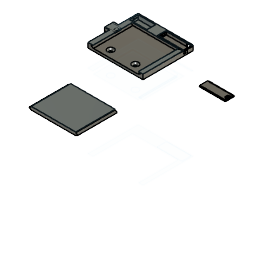
3d molde Home assistnt tablat (Autodesk Fusion 360 design; units mm, degrees)
part number: 2026-03-25-17-44-52-622
Autodesk Fusion 360 part; units mm, degrees
note: some values were not read from the file. Chosen so that the rebuilt part matches the saved one: which bodies a step acts on; which face or edge a step refers to.
(part 1 of 2)
sketch "Skizze1" plane through (0, 0, 0) normal (0, 0, 1) x (1, 0, 0)
  line L0 (0, 0) -> (242, 0)
  line L1 (242, 0) -> (242, 166)
  line L2 (242, 166) -> (0, 166)
  line L3 (0, 166) -> (0, 0)
  dimension "d1" = 242
  dimension "d2" = 166
  constraint horizontal L0
  constraint vertical L1
  constraint horizontal L2
  constraint vertical L3
  constraint coincident L0.start L3.end
  measures "d1" distance of L0.start L0.end
  measures "d2" distance of L0.start L2.end
extrude "Extrusion1" add sketch "Skizze1" along normal blind 7.5 makes body 1
fillet "Abrundung1" radius 7.5 4 edges at (0, 0, 3.75) (242, 0, 3.75) (242, 166, 3.75) (0, 166, 3.75) on bodies 1
sketch "Skizze2" plane through (0, 0, 7.5) normal (0, 0, 1) x (-1, 0, 0)
  arc A0 (-7.5, -166) -> (0, -158.5) centre (-7.5, -158.5) ccw
  line L0 (0, -158.5) -> (0, -7.5)
  arc A1 (0, -7.5) -> (-7.5, 0) centre (-7.5, -7.5) ccw
  line L1 (-7.5, 0) -> (-234.5, 0)
  arc A2 (-234.5, 0) -> (-242, -7.5) centre (-234.5, -7.5) ccw
  line L2 (-242, -7.5) -> (-242, -158.5)
  arc A3 (-242, -158.5) -> (-234.5, -166) centre (-234.5, -158.5) ccw
  line L3 (-234.5, -166) -> (-7.5, -166)
  line L4 (-199.0459, -30) -> (-43.7756, -30)
  line L5 (-43.7756, -30) -> (-43.7756, -136.2508)
  line L6 (-43.7756, -136.2508) -> (-199.0459, -136.2508)
  line L7 (-199.0459, -136.2508) -> (-199.0459, -30)
  constraint horizontal L4
  constraint vertical L5
  constraint horizontal L6
  constraint vertical L7
extrude "Extrusion2" add sketch "Skizze2" along normal blind 10 contours L4 L5 L6 L7 bodies 1
sketch "Skizze3" plane through (0, 166, 0) normal (0, 1, 0) x (-1, 0, 0)
  line L0 (-7.5, 0) -> (-7.5, 7.5)
  line L1 (-7.5, 7.5) -> (-234.5, 7.5)
  line L2 (-234.5, 7.5) -> (-234.5, 0)
  line L3 (-234.5, 0) -> (-7.5, 0)
  line L4 (-259.0579, 7.5) -> (20, 7.5)
  line L5 (20, 7.5) -> (20, -40)
  line L6 (20, -40) -> (-259.0579, -40)
  line L7 (-259.0579, -40) -> (-259.0579, 7.5)
  constraint horizontal L4
  constraint vertical L5
  constraint horizontal L6
  constraint vertical L7
extrude "Extrusion3" cut sketch "Skizze3" against normal blind 170 bodies 1
sketch "Skizze4" plane through (0, 0, 17.5) normal (0, 0, 1) x (-1, 0, 0)
  line L0 (-199.0459, -136.2508) -> (-43.7756, -136.2508)
  line L1 (-43.7756, -136.2508) -> (-43.7756, -30)
  line L2 (-43.7756, -30) -> (-199.0459, -30)
  line L3 (-199.0459, -30) -> (-199.0459, -136.2508)
  line L4 (40, -30) -> (140, -30)
  line L5 (140, -30) -> (140, -110)
  line L6 (140, -110) -> (40, -110)
  line L7 (40, -110) -> (40, -30)
  dimension "d15" = 100
  dimension "d16" = 80
  constraint horizontal L4
  constraint vertical L5
  constraint horizontal L6
  constraint vertical L7
  measures "d15" distance of L4.start L4.end
  measures "d16" distance of L4.start L6.end
extrude "Extrusion4" add sketch "Skizze4" against normal blind 5 separate body contours L4 L5 L6 L7 makes body 2
extrude "Extrusion5" add 1 faces at (-73.3333, 56.6667, 17.5) along direction (0, 0, 1) blind 10 on bodies 2 bodies 2
sketch "Skizze5" plane through (0, 0, 27.5) normal (0, 0, 1) x (-1, 0, 0)
  line L0 (40, -110) -> (140, -110)
  line L1 (140, -110) -> (140, -30)
  line L2 (140, -30) -> (40, -30)
  line L3 (40, -30) -> (40, -110)
extrude "Extrusion6" cut sketch "Skizze5" against normal blind 10 bodies 2
extrude "Extrusion7" add 1 faces at (-73.3333, 56.6667, 17.5) along direction (0, 0, 1) blind 0.5 on bodies 2 bodies 2
sketch "Skizze6" plane through (0, 30, 0) normal (0, -1, 0) x (1, 0, 0)
  line L0 (-140, 18) -> (-140, 12.5)
  line L1 (-140, 12.5) -> (-40, 12.5)
  line L2 (-40, 12.5) -> (-40, 18)
  line L3 (-40, 18) -> (-140, 18)
  line L4 (-140, 15.25) -> (-134.9888, 18)
  line L5 (-140, 18) -> (-140, 12.5)
  line L6 (-135.0937, 12.5) -> (-140, 15.25)
  line L7 (-140, 12.5) -> (-135.0937, 12.5)
  line L8 (-140, 18) -> (-134.9888, 18)
  line L9 (-44.7811, 18) -> (-40, 15.25)
  line L10 (-44.886, 12.5) -> (-40, 15.25)
  line L11 (-44.886, 12.5) -> (-40, 12.5)
  line L12 (-40, 12.5) -> (-40, 18)
  line L13 (-40, 18) -> (-44.7811, 18)
  constraint midpoint L0 L4.start
  constraint coincident L3 L4.end
  constraint coincident L0.start L3.end
  constraint coincident L0.end L1.start
  constraint coincident L1 L6.start
  constraint coincident L3 L9.start
  constraint midpoint L2 L9.end
  constraint coincident L1 L10.start
  constraint coincident L1.end L2.start
  constraint coincident L2.end L3.start
extrude "Extrusion8" cut sketch "Skizze6" against normal blind 90 contours L0 L3 L4 L5 L8 | L0 L1 L5 L6 L7 | L2 L3 L9 L12 L13 | L1 L2 L10 L11 L12 bodies 2
move_body "Verschieben1" bodies 2 to x (1, 0, 0) y (0, 1, 0) z (0, 0, 1) at (210, -110, 0)
move_body "Verschieben2" bodies 2 to x (1, 0, 0) y (0, 1, 0) z (0, 0, 1) at (-10, 0, 0)
sketch "Skizze7" plane through (0, 0, 17.5) normal (0, 0, 1) x (-1, 0, 0)
  line L0 (-199.0459, -136.2508) -> (-43.7756, -136.2508)
  line L1 (-43.7756, -136.2508) -> (-43.7756, -30)
  line L2 (-43.7756, -30) -> (-199.0459, -30)
  line L3 (-199.0459, -30) -> (-199.0459, -136.2508)
  line L4 (-175.238, -30) -> (-199.0459, -30)
  line L5 (-199.0459, -136.2508) -> (-175, -136.2508)
  line L6 (-175.238, -30) -> (-175, -136.2508)
  line L7 (-199.0459, -30) -> (-199.0459, -136.2508)
  constraint coincident L2 L4.start
  constraint coincident L2.end L3.start
  constraint coincident L0.start L3.end
  constraint coincident L0 L5.end
extrude "Extrusion9" cut sketch "Skizze7" against normal blind 150 contours L0 L2 L3 L4 L5 L6 L7 bodies 1
sketch "Skizze8" plane through (0, 0, 17.5) normal (0, 0, 1) x (-1, 0, 0)
  line L0 (-175.238, -30) -> (-175, -136.2508)
  line L1 (-175, -136.2508) -> (-43.7756, -136.2508)
  line L2 (-43.7756, -136.2508) -> (-43.7756, -30)
  line L3 (-43.7756, -30) -> (-175.238, -30)
  line L4 (-180, -130) -> (-40, -130)
  line L5 (-40, -130) -> (-40, -140)
  line L6 (-40, -140) -> (-180, -140)
  line L7 (-180, -140) -> (-180, -130)
  constraint horizontal L4
  constraint vertical L5
  constraint horizontal L6
  constraint vertical L7
extrude "Extrusion10" cut sketch "Skizze8" against normal blind 20 contours L0 L1 L2 L4 | L0 L1 L2 L4 L5 L6 L7 bodies 1
extrude "Extrusion11" cut 1 faces at (95.0105, 0, 14.3333) along direction (0, 1, 0) blind 120 on bodies 2 bodies 1
move_body "Verschieben3" bodies 2 to x (1, 0, 0) y (0, 1, 0) z (0, 0, 1) at (0, 25, 0)
sketch "Skizze9" plane through (0, 0, 12.5) normal (0, 0, 1) x (-1, 0, 0)
  line L0 (-64.9063, -30) -> (-155.114, -30)
  line L1 (-155.114, -30) -> (-155.114, -120)
  line L2 (-155.114, -120) -> (-64.9063, -120)
  line L3 (-64.9063, -120) -> (-64.9063, -30)
  line L4 (-135, -45) -> (-175, -45)
  line L5 (-45, -45) -> (-85, -45)
  dimension "d33" = 40
  constraint perpendicular L3 L5
  constraint horizontal L4
  measures "d33" distance of L5.start L5.end
hole "Bohrung1" at (85, 45, 12.5) at (135, 45, 12.5) direction (0, 0, -1) diameter 6 depth 55 tip angle 118 countersink diameter 13 countersink angle 90 bodies 1
extrude "Extrusion12" add 1 faces at (125.1008, 120, 15.8333) along direction (0, -1, 0) blind 10 on bodies 1 bodies 1
move_body "Verschieben4" bodies 2 to x (1, 0, 0) y (0, 1, 0) z (0, 0, 1) at (0, 0, -50)
extrude "Extrusion13" cut 1 faces at (87.5217, 130, 10.8333) along direction (0, -1, 0) blind 10 on bodies 1 bodies 1
extrude "Extrusion14" cut 1 faces at (175.1633, 63.3333, 14.1667) along direction (-0.999997, -0.00224, 0) blind 10 on bodies 1 bodies 1
extrude "Extrusion15" cut 1 faces at (43.7756, 60, 10.8333) along direction (1, 0, 0) blind 10 on bodies 1 bodies 1
move_body "Verschieben5" bodies 2 to x (1, 0, 0) y (0, 1, 0) z (0, 0, 1) at (0, -20, 50)
extrude "Extrusion16" add 1 faces at (127.9494, 120, 10.8333) along direction (0, 1, 0) blind 10 on bodies 1 bodies 1
sketch "Skizze10" plane through (0, 0, 17.5) normal (0, 0, 1) x (-1, 0, 0)
extrude "Extrusion17" add 1 faces at (127.9494, 130, 10.8333) along direction (0, 1, 0) blind 2 on bodies 1 bodies 1
sketch "Skizze11" plane through (0, 0, 17.5) normal (0, 0, 1) x (-1, 0, 0)
  line L0 (-162.2484, -111.5795) -> (-132.2484, -111.5795)
  line L1 (-132.2484, -111.5795) -> (-132.2484, -130.0795)
  line L2 (-132.2484, -130.0795) -> (-162.2484, -130.0795)
  line L3 (-162.2484, -130.0795) -> (-162.2484, -111.5795)
  dimension "d51" = 30
  dimension "d52" = 18.5
  constraint horizontal L0
  constraint vertical L1
  constraint horizontal L2
  constraint vertical L3
  measures "d51" distance of L0.start L0.end
  measures "d52" distance of L0.start L2.end
sketch "Skizze12" plane through (0, 0, 17.5) normal (0, 0, 1) x (-1, 0, 0)
extrude "Extrusion18" cut sketch "Skizze11" against normal blind 8 bodies 1
sketch "Skizze13" plane through (0, 132, 0) normal (0, 1, 0) x (-1, 0, 0)
  line L0 (-53.7756, 7.5) -> (-53.7756, 17.5)
  line L1 (-53.7756, 17.5) -> (-165.0364, 17.5)
  line L2 (-165.0364, 17.5) -> (-165.0364, 7.5)
  line L3 (-165.0364, 7.5) -> (-53.7756, 7.5)
  line L4 (-162, 15) -> (-153, 15)
  line L5 (-153, 15) -> (-153, 12)
  line L6 (-153, 12) -> (-162, 12)
  line L7 (-162, 12) -> (-162, 15)
  dimension "d55" = 9
  dimension "d56" = 3
  constraint horizontal L4
  constraint vertical L5
  constraint horizontal L6
  constraint vertical L7
  measures "d55" distance of L4.start L4.end
  measures "d56" distance of L4.start L6.end
extrude "Extrusion19" cut sketch "Skizze13" against normal blind 5 contours L4 L5 L6 L7 bodies 1
extrude "Extrusion20" cut 1 faces at (156, 131.3598, 12) along direction (0, 0, -1) blind 3 on bodies 1 bodies 1
extrude "Extrusion21" add 1 faces at (125.1497, -48.3333, 18) along direction (0, 0, 1) blind 1 on bodies 2 bodies 2
extrude "Extrusion22" cut 1 faces at (156.8126, -48.3333, 17.0833) along direction (-0.498592, 0, -0.866837) blind 0.2 on bodies 2 bodies 2
extrude "Extrusion23" cut 1 faces at (156.6751, -21.6667, 13.3786) along direction (-0.490484, 0, 0.87145) blind 0.2 on bodies 2 bodies 2
extrude "Extrusion24" cut 1 faces at (63.2709, -48.3333, 13.4167) along direction (0.488937, 0, 0.872319) blind 0.2 on bodies 2 bodies 2
extrude "Extrusion25" cut 1 faces at (63.4097, -21.6667, 17.1211) along direction (0.481091, 0, -0.876671) blind 0.2 on bodies 2 bodies 2
sketch "Skizze14" plane through (0, 0, 19) normal (0, 0, 1) x (-1, 0, 0)
  line L0 (-155.2189, 75) -> (-155.2189, -5)
  line L1 (-155.2189, -5) -> (-65.0112, -5)
  line L2 (-65.0112, -5) -> (-65.0112, 75)
  line L3 (-65.0112, 75) -> (-155.2189, 75)
  line L4 (-4.4649, 104.0889) -> (237.5351, 104.0889)
  line L5 (237.5351, 104.0889) -> (237.5351, -61.9111)
  line L6 (237.5351, -61.9111) -> (-4.4649, -61.9111)
  line L7 (-4.4649, -61.9111) -> (-4.4649, 104.0889)
  dimension "d71" = 242
  dimension "d72" = 166
  constraint horizontal L4
  constraint vertical L5
  constraint horizontal L6
  constraint vertical L7
  measures "d71" distance of L4.start L4.end
  measures "d72" distance of L4.start L6.end
sketch "Skizze15" plane through (0, 0, 26.7) normal (0, 0, 1) x (-1, 0, 0)
  arc A0 (3.0351, 104.0889) -> (-4.4649, 96.5889) centre (3.0351, 96.5889) ccw
  line L0 (-4.4649, 96.5889) -> (-4.4649, -54.4111)
  arc A1 (-4.4649, -54.4111) -> (3.0351, -61.9111) centre (3.0351, -54.4111) ccw
  line L1 (3.0351, -61.9111) -> (230.0351, -61.9111)
  arc A2 (230.0351, -61.9111) -> (237.5351, -54.4111) centre (230.0351, -54.4111) ccw
  line L2 (237.5351, -54.4111) -> (237.5351, 96.5889)
  arc A3 (237.5351, 96.5889) -> (230.0351, 104.0889) centre (230.0351, 96.5889) ccw
  line L3 (230.0351, 104.0889) -> (3.0351, 104.0889)
  line L4 (9.6749, 27.3289) -> (3.4349, 27.3289)
  line L5 (3.4349, 27.3289) -> (3.4351, 21.0889)
  line L6 (9.6749, 27.3289) -> (15.9149, 27.3289)
  line L7 (15.9149, 27.3289) -> (15.9149, 14.8489)
  line L8 (15.9149, 14.8489) -> (3.4349, 14.8485)
  line L9 (3.4349, 14.8485) -> (3.4349, 27.3289)
  dimension "d80" = 6.24
  dimension "d81" = 6.24
  dimension "d82" = 12.48
  constraint perpendicular L4 L7
  constraint perpendicular L5 L8
  constraint perpendicular L4 L9
  measures "d80" distance of L4.start L4.end
  measures "d81" distance of L4.start L6.end
  measures "d82" distance of L6.end L7.end
sketch "Skizze16" plane through (0, 0, 27.2) normal (0, 0, 1) x (-1, 0, 0)
  line L0 (15.4149, 15.3489) -> (15.4149, 26.8289)
  line L1 (15.4149, 26.8289) -> (3.9349, 26.8289)
  line L2 (3.9349, 26.8289) -> (3.9349, 15.3485)
  line L3 (3.9349, 15.3485) -> (15.4149, 15.3489)
  circle A0 centre (9.6749, 21.0887) radius 1.75
  dimension "d87" = 3.5
  measures "d87" diameter of A0
sketch "Skizze17" plane through (-237.5351, 0, 0) normal (-1, 0, 0) x (0, -1, 0)
  line L0 (96.5889, 19) -> (96.5889, 26.7)
  line L1 (96.5889, 26.7) -> (-54.4111, 26.7)
  line L2 (-54.4111, 26.7) -> (-54.4111, 19)
  line L3 (-54.4111, 19) -> (96.5889, 19)
  line L4 (18.0776, 22.85) -> (18.0776, 21.5)
  line L5 (23.9968, 22.85) -> (24, 21.5)
  line L6 (23.9968, 22.85) -> (23.7, 23.2)
  line L7 (18.0776, 22.85) -> (18.4903, 23.2)
  line L8 (21.0889, 23.2) -> (23.7, 23.2)
  line L9 (18.4903, 23.2) -> (21.0889, 23.2)
  line L10 (18.0776, 21.5) -> (24, 21.5)
  constraint perpendicular L6 L7
sketch "Skizze18" plane through (-232.5351, 0, 0) normal (-1, 0, 0) x (0, -1, 0)
  line L0 (18.0776, 22.85) -> (18.0776, 21.5)
  line L1 (18.0776, 21.5) -> (24, 21.5)
  line L2 (24, 21.5) -> (23.9968, 22.85)
  line L3 (23.9968, 22.85) -> (23.7, 23.2)
  line L4 (23.7, 23.2) -> (21.0889, 23.2)
  line L5 (21.0889, 23.2) -> (18.4903, 23.2)
  line L6 (18.4903, 23.2) -> (18.0776, 22.85)
  line L7 (19, 22.5) -> (23, 22.5)
  line L8 (23, 22.5) -> (23, 22)
  line L9 (23, 22) -> (19, 22)
  line L10 (19, 22) -> (19, 22.5)
  constraint horizontal L7
  constraint vertical L8
  constraint horizontal L9
  constraint vertical L10
move_body "Verschieben6" bodies 2 to x (1, 0, 0) y (0, 1, 0) z (0, 0, 1) at (-225, 10, 25)
move_body "Verschieben7" bodies 2 to x (1, 0, 0) y (0, 1, 0) z (0, 0, 1) at (0, 5, 0)
sketch "Skizze19" plane through (0, 0, 44) normal (0, 0, 1) x (-1, 0, 0)
move_body "Verschieben8" [no effect]
move_body "Verschieben9" bodies 1 to x (1, 0, 0) y (0, 1, 0) z (0, 0, 1) at (-75, 0, 0)
move_body "Verschieben10" bodies 1 to x (1, 0, 0) y (0, 1, 0) z (0, 0, 1) at (-140, 0, 50)
move_body "Verschieben11" bodies 1 to x (1, 0, 0) y (0, 1, 0) z (0, 0, 1) at (120, 0, -70)
move_body "Verschieben12" bodies 2 to x (1, 0, 0) y (0, 1, 0) z (0, 0, 1) at (135, 14, -50)
move_body "Verschieben13" bodies 2 to x (1, 0, 0) y (0, 1, 0) z (0, 0, 1) at (-5, 0, 5)
extrude "Extrusion31" cut 1 faces at (37.2484, 117.7462, -5.1667) along direction (-1, 0, 0) blind 20 on bodies 1 bodies 1
extrude "Extrusion32" cut 1 faces at (30.8322, 130.0795, -6) along direction (0, 1, 0) blind 0.5 on bodies 1 bodies 1
move_body "Verschieben14" bodies 2 to x (1, 0, 0) y (0, 1, 0) z (0, 0, 1) at (0, -50, 0)
sketch "Skizze20" plane through (17.2484, 0, 0) normal (1, 0, 0) x (0, 1, 0)
  line L0 (130.5795, -2.5) -> (111.5795, -2.5)
  line L1 (111.5795, -2.5) -> (111.5795, -10.5)
  line L2 (111.5795, -10.5) -> (130.5795, -10.5)
  line L3 (130.5795, -10.5) -> (130.5795, -2.5)
  circle A0 centre (121.0795, -6.5) radius 1.5
  dimension "d106" = 3
  measures "d106" diameter of A0
sketch "Skizze21" plane through (0, 0, -2.5) normal (0, 0, 1) x (-1, 0, 0)
  line L0 (41.2244, -132) -> (41.2244, -30)
  line L1 (41.2244, -30) -> (30.8999, -30)
  line L2 (30.8999, -30) -> (30.8999, -110)
  line L3 (30.8999, -110) -> (-61.0882, -110)
  line L4 (-61.0882, -110) -> (-61.0882, -30)
  line L5 (-61.0882, -30) -> (-70.2379, -30)
  line L6 (-70.2379, -30) -> (-70.0364, -120)
  line L7 (-70.0364, -120) -> (-70.0364, -132)
  line L8 (-70.0364, -132) -> (41.2244, -132)
  line L9 (-17.2484, -111.5795) -> (-17.2484, -130.5795)
  line L10 (-17.2484, -130.5795) -> (-67.2484, -130.5795)
  line L11 (-67.2484, -130.5795) -> (-67.2484, -111.5795)
  line L12 (-67.2484, -111.5795) -> (-17.2484, -111.5795)
sketch "Skizze22" plane through (0, 30, 0) normal (0, -1, 0) x (1, 0, 0)
  line L0 (-41.2244, -2.5) -> (-41.2244, -12.5)
  line L1 (-41.2244, -12.5) -> (70.2379, -12.5)
  line L2 (70.2379, -12.5) -> (70.2379, -2.5)
  line L3 (70.2379, -2.5) -> (61.0882, -2.5)
  line L4 (61.0882, -2.5) -> (65, -4.75)
  line L5 (65, -4.75) -> (60.114, -7.5)
  line L6 (60.114, -7.5) -> (-30.0937, -7.5)
  line L7 (-30.0937, -7.5) -> (-35, -4.75)
  line L8 (-35, -4.75) -> (-30.8999, -2.5)
  line L9 (-30.8999, -2.5) -> (-41.2244, -2.5)
  circle A0 centre (-37.199, -6.5) radius 1.5
  dimension "d108" = 3
  measures "d108" diameter of A0
extrude "Extrusion33" cut sketch "Skizze22" against normal blind 99 contours A0 bodies 1
hole "Bohrung2" at (17.2484, 121.0795, -6.5) direction (-1, 0, 0) diameter 3 depth 56.5 tip angle 180 bodies 1
sketch "Skizze23" plane through (0, 0, -2.5) normal (0, 0, 1) x (-1, 0, 0)
  line L0 (24, -115) -> (38, -115)
  line L1 (38, -115) -> (38, -129)
  line L2 (38, -129) -> (24, -129)
  line L3 (24, -129) -> (24, -115)
  constraint horizontal L0
  constraint vertical L1
  constraint horizontal L2
  constraint vertical L3
extrude "Extrusion34" cut sketch "Skizze23" against normal blind 5.5 bodies 1
sketch "Skizze24" plane through (0, 0, -2.5) normal (0, 0, 1) x (-1, 0, 0)
move_body "Verschieben15" bodies 1 to x (1, 0, 0) y (0, 1, 0) z (0, 0, 1) at (0, 0, 150)
sketch "Skizze25" plane through (0, 0, 142) normal (0, 0, 1) x (-1, 0, 0)
  line L0 (37.199, -115) -> (24, -115)
  line L1 (24, -115) -> (24, -121.0795)
  line L2 (24, -121.0795) -> (24, -129)
  line L3 (24, -129) -> (38, -129)
  line L4 (38, -129) -> (38, -121.0795)
  line L5 (38, -121.0795) -> (38, -115)
  line L6 (38, -115) -> (37.199, -115)
  line L7 (24, -122.719) -> (38, -122.719)
  line L8 (38, -122.719) -> (38, -129)
  line L9 (38, -129) -> (24, -129)
  line L10 (24, -129) -> (24, -122.719)
  line L11 (24, -120) -> (35.3869, -115)
  line L12 (27.3055, -122.719) -> (38, -115)
  constraint horizontal L7
  constraint vertical L8
  constraint horizontal L9
  constraint vertical L10
  constraint coincident L3.end L4.start
  constraint coincident L2 L7.start
  constraint coincident L1 L11.start
  constraint coincident L0 L11.end
  constraint coincident L7 L12.start
  constraint coincident L5.end L6.start
extrude "Extrusion35" add sketch "Skizze25" along normal blind 5.5 contours L0 L1 L11 | L4 L5 L7 L12 | L2 L3 L4 L7 L8 L9 L10 bodies 1
sketch "Skizze26" plane through (0, 0, 147.5) normal (0, 0, 1) x (-1, 0, 0)
  line L0 (24, -122.719) -> (24, -120)
  line L1 (24, -120) -> (35.3869, -115)
  line L2 (35.3869, -115) -> (38, -115)
  line L3 (38, -115) -> (27.3055, -122.719)
  line L4 (27.3055, -122.719) -> (24, -122.719)
  line L5 (41.2244, -132) -> (41.2244, -30)
  line L6 (41.2244, -30) -> (30.8999, -30)
  line L7 (30.8999, -30) -> (30.8999, -110)
  line L8 (30.8999, -110) -> (-61.0882, -110)
  line L9 (-61.0882, -110) -> (-61.0882, -30)
  line L10 (-61.0882, -30) -> (-70.2379, -30)
  line L11 (-70.2379, -30) -> (-70.0364, -120)
  line L12 (-70.0364, -120) -> (-70.0364, -132)
  line L13 (-70.0364, -132) -> (41.2244, -132)
  line L14 (-17.2484, -111.5795) -> (-17.2484, -130.5795)
  line L15 (-17.2484, -130.5795) -> (-67.2484, -130.5795)
  line L16 (-67.2484, -130.5795) -> (-67.2484, -111.5795)
  line L17 (-67.2484, -111.5795) -> (-17.2484, -111.5795)
  line L18 (27.3055, -122.719) -> (30.5, -122.719)
  line L19 (30.5, -122.719) -> (38.5, -115)
  line L20 (38.5, -115) -> (38, -115)
  line L21 (27.3055, -122.719) -> (38, -115)
  constraint coincident L3.end L4.start
  constraint parallel L4 L18
  constraint coincident L2.end L3.start
  constraint parallel L2 L20
extrude "Extrusion36" cut sketch "Skizze26" against normal blind 5.5 contours L3 L18 L19 L20 L21 bodies 1
sketch "Skizze27" plane through (-48.0542, 109.4378, 0) normal (-0.402048, 0.915618, 0) x (-0.915618, -0.402048, 0)
  line L0 (-26.271, 142) -> (-13.8346, 142)
  line L1 (-13.8346, 142) -> (-13.8346, 147.5)
  line L2 (-13.8346, 147.5) -> (-26.271, 147.5)
  line L3 (-26.271, 147.5) -> (-26.271, 144.5415)
  line L4 (-26.271, 144.5415) -> (-26.271, 142.4585)
  line L5 (-26.271, 142.4585) -> (-26.271, 142)
  line L6 (-26.271, 145.5318) -> (-10.1512, 145.5318)
  line L7 (-10.1512, 145.5318) -> (-10.1512, 147.4938)
  line L8 (-10.1512, 147.4938) -> (-26.271, 147.5)
  line L9 (-26.271, 145.5318) -> (-26.271, 147.5)
  constraint coincident L3 L6.start
  constraint perpendicular L1 L6
  constraint perpendicular L6 L7
  constraint coincident L2.end L3.start
extrude "Extrusion37" add sketch "Skizze27" along normal blind 6 contours L1 L3 L6 L8 L9 bodies 1
sketch "Skizze28" plane through (24.0542, 10.5622, 0) normal (0.915618, 0.402048, 0) x (-0.402048, 0.915618, 0)
  line L0 (122.493, 145.5318) -> (122.493, 147.5)
  line L1 (122.493, 147.5) -> (119.5234, 147.5)
  line L2 (119.5234, 147.5) -> (119.5234, 145.5318)
  line L3 (119.5234, 145.5318) -> (122.493, 145.5318)
extrude "Extrusion38" add sketch "Skizze28" along normal blind 3.5 bodies 1
sketch "Skizze29" plane through (12.6672, 5.5622, 0) normal (-0.915618, -0.402048, 0) x (0.402048, -0.915618, 0)
  line L0 (-121.8277, 147.4952) -> (-121.8277, 145.5318)
  line L1 (-121.8277, 145.5318) -> (-119.5234, 145.5318)
  line L2 (-119.5234, 145.5318) -> (-119.5234, 147.4952)
  line L3 (-119.5234, 147.4952) -> (-121.8277, 147.4952)
extrude "Extrusion39" add sketch "Skizze29" along normal blind 3 bodies 1
sketch "Skizze30" plane through (-41.2244, 0, 0) normal (-1, 0, 0) x (0, -1, 0)
  line L0 (-132, 137.5) -> (-30, 137.5)
  line L1 (-30, 137.5) -> (-30, 147.5)
  line L2 (-30, 147.5) -> (-132, 147.5)
  line L3 (-132, 147.5) -> (-132, 137.5)
  circle A0 centre (-82.7183, 143.5) radius 1.75
  dimension "d127" = 3.5
  measures "d127" diameter of A0
extrude "Extrusion40" cut sketch "Skizze30" against normal blind 5.5 contours A0 bodies 1
sketch "Skizze31" plane through (-41.2244, 0, 0) normal (-1, 0, 0) x (0, -1, 0)
  circle A0 centre (-82.7183, 143.5) radius 1.75
  line L0 (-132, 137.5) -> (-30, 137.5)
  line L1 (-30, 137.5) -> (-30, 147.5)
  line L2 (-30, 147.5) -> (-132, 147.5)
  line L3 (-132, 147.5) -> (-132, 137.5)
  line L4 (-81, 145.5) -> (-78.6246, 145.5)
  line L5 (-78.6246, 145.5) -> (-78.6246, 141.4531)
  line L6 (-78.6246, 141.4531) -> (-81, 141.4531)
  line L7 (-81, 141.4531) -> (-81, 145.5)
  constraint horizontal L4
  constraint vertical L5
  constraint horizontal L6
  constraint vertical L7
extrude "Extrusion41" add sketch "Skizze31" against normal blind 5 contours A0 L4 L5 L6 L7 bodies 1
sketch "Skizze32" plane through (-41.2244, 0, 0) normal (-1, 0, 0) x (0, -1, 0)
  circle A0 centre (-82.7183, 143.5) radius 1.75
  line L0 (-132, 137.5) -> (-30, 137.5)
  line L1 (-30, 137.5) -> (-30, 147.5)
  line L2 (-30, 147.5) -> (-132, 147.5)
  line L3 (-132, 147.5) -> (-132, 137.5)
  line L4 (-78.4813, 147.5) -> (-30, 147.5)
  line L5 (-30, 147.5) -> (-30, 137.5)
  line L6 (-30, 137.5) -> (-78.4813, 137.5)
  line L7 (-78.4813, 137.5) -> (-78.4813, 147.5)
  constraint horizontal L4
  constraint vertical L5
  constraint horizontal L6
  constraint vertical L7
  constraint coincident L0.end L1.start
  constraint coincident L2 L4.start
extrude "Extrusion42" add sketch "Skizze32" against normal blind 6 contours L0 L1 L2 L4 L5 L6 L7 bodies 1
sketch "Skizze33" plane through (70.3048, 0.1575, 0) normal (0.999997, 0.00224, 0) x (-0.00224, 0.999997, 0)
  line L0 (29.8426, 147.5) -> (29.8426, 137.5)
  line L1 (29.8426, 137.5) -> (119.8428, 137.5)
  line L2 (119.8428, 137.5) -> (119.8428, 147.5)
  line L3 (119.8428, 147.5) -> (29.8426, 147.5)
  line L4 (111.5, 147.5) -> (130.2493, 147.5)
  line L5 (130.2493, 147.5) -> (130.2493, 145.6301)
  line L6 (130.2493, 145.6301) -> (111.5, 145.6301)
  line L7 (111.5, 145.6301) -> (111.5, 147.5)
  constraint horizontal L4
  constraint vertical L5
  constraint horizontal L6
  constraint vertical L7
  constraint coincident L3 L4.start
extrude "Extrusion43" cut sketch "Skizze33" against normal blind 52.5 contours L2 L3 L4 L6 L7 | L2 L4 L5 L6 bodies 1
sketch "Skizze34" plane through (70.0364, 0, 0) normal (1, 0, 0) x (0, 1, 0)
  line L0 (120, 147.5) -> (120, 145.6301)
  line L1 (120, 145.6301) -> (120, 137.5)
  line L2 (120, 137.5) -> (132, 137.5)
  line L3 (132, 137.5) -> (132, 147.5)
  line L4 (132, 147.5) -> (120, 147.5)
  line L5 (120, 145.6301) -> (130.5, 145.6301)
  line L6 (130.5, 145.6301) -> (130.5, 147.5)
  line L7 (130.5, 147.5) -> (120, 147.5)
  line L8 (120, 147.5) -> (120, 145.6301)
  constraint horizontal L5
  constraint vertical L6
  constraint horizontal L7
  constraint vertical L8
  constraint coincident L4 L6.end
  constraint coincident L0.end L1.start
extrude "Extrusion44" cut sketch "Skizze34" against normal blind 52.5 contours L0 L4 L5 L6 L7 L8 bodies 1
sketch "Skizze35" plane through (17.2484, 0, 0) normal (1, 0, 0) x (0, 1, 0)
  circle A0 centre (121.0795, 143.5) radius 1.5
  line L0 (130.5795, 147.5) -> (111.5795, 147.5)
  line L1 (111.5795, 147.5) -> (111.5795, 139.5)
  line L2 (111.5795, 139.5) -> (130.5795, 139.5)
  line L3 (130.5795, 139.5) -> (130.5795, 147.5)
  line L4 (111.6591, 147.5) -> (113.1591, 147.5)
  line L5 (113.1591, 147.5) -> (113.1591, 147)
  line L6 (113.1591, 147) -> (111.6591, 147)
  line L7 (111.6591, 147) -> (111.6591, 147.5)
  line L8 (130.5, 147.5) -> (129, 147.5)
  line L9 (129, 147.5) -> (129, 147)
  line L10 (129, 147) -> (130.5, 147)
  line L11 (130.5, 147) -> (130.5, 147.5)
  dimension "d138" = 1.5
  dimension "d139" = 0.5
  dimension "d140" = 1.5
  dimension "d141" = 0.5
  constraint horizontal L4
  constraint vertical L5
  constraint horizontal L6
  constraint vertical L7
  constraint coincident L0 L4.start
  constraint horizontal L8
  constraint vertical L9
  constraint horizontal L10
  constraint vertical L11
  constraint coincident L0 L8.start
  measures "d138" distance of L4.start L4.end
  measures "d139" distance of L4.start L6.end
  measures "d140" distance of L8.start L8.end
  measures "d141" distance of L8.start L10.end
extrude "Extrusion45" add sketch "Skizze35" along normal blind 53 contours L0 L8 L9 L10 L11 | L0 L4 L5 L6 L7 bodies 1
extrude "Extrusion46" add 1 faces at (52.5817, 111.6591, 147.1667) along direction (0, -1, 0) blind 0.1 on bodies 1 bodies 1
extrude "Extrusion47" add 1 faces at (23.3607, 111.5591, 147.3333) along direction (0, -1, 0) blind 0.1 on bodies 1 bodies 1
extrude "Extrusion48" add 1 faces at (50.5817, 130.5, 147.3333) along direction (0, 1, 0) blind 0.1 on bodies 1 bodies 1
extrude "Extrusion49" cut 1 faces at (70.107, 130.5, 147.3333) along direction (0, -1, 0) blind 26 on bodies 1 bodies 1
extrude "Extrusion50" add 1 faces at (70.0364, 109.7721, 147.3333) along direction (1, 0, 0) blind 0.0347 on bodies 1 bodies 1
sketch "Skizze36" plane through (17.2484, 0, 0) normal (1, 0, 0) x (0, 1, 0)
  line L0 (130.5795, 147) -> (129, 147)
  line L1 (129, 147) -> (129, 147.5)
  line L2 (129, 147.5) -> (113.1591, 147.5)
  line L3 (113.1591, 147.5) -> (113.1591, 147)
  line L4 (113.1591, 147) -> (111.5795, 147)
  line L5 (111.5795, 147) -> (111.5795, 139.5)
  line L6 (111.5795, 139.5) -> (130.5795, 139.5)
  line L7 (130.5795, 139.5) -> (130.5795, 147)
  circle A0 centre (121.0795, 143.5) radius 1.5
  line L8 (111.7, 146.9) -> (113.2, 146.9)
  line L9 (113.2, 146.9) -> (113.2, 147.5)
  line L10 (111.7, 145.7) -> (111.7, 146.9)
  line L11 (111.7, 145.7) -> (130.4, 145.7)
  line L12 (130.4, 145.7) -> (130.4, 146.9)
  line L13 (130.4, 146.9) -> (128.9, 146.9)
  line L14 (128.9, 146.9) -> (128.9, 147.5)
  line L15 (113.2, 147.5) -> (128.9, 147.5)
  constraint perpendicular L5 L8
  constraint coincident L2 L9.end
  constraint perpendicular L2 L9
  constraint perpendicular L8 L10
  constraint perpendicular L7 L11
  constraint perpendicular L11 L12
  constraint perpendicular L7 L13
  constraint coincident L2 L14.end
  constraint perpendicular L2 L14
extrude "Extrusion51" add sketch "Skizze36" along normal blind 130 contours L2 L8 L9 L10 L11 L12 L13 L14 L15 bodies 1
sketch "Skizze37" plane through (0, 0, 147.5) normal (0, 0, 1) x (-1, 0, 0)
  line L0 (25.1939, -122.719) -> (24, -120)
  line L1 (24, -120) -> (35.3869, -115)
  line L2 (35.3869, -115) -> (38.5, -115)
  line L3 (38.5, -115) -> (30.5, -122.719)
  line L4 (30.5, -122.719) -> (25.1939, -122.719)
  line L5 (-70.0711, -113.1591) -> (-17.2484, -113.1591)
  line L6 (-17.2484, -113.1591) -> (-17.2484, -113.2)
  line L7 (-17.2484, -113.2) -> (-147.2484, -113.2)
  line L8 (-147.2484, -113.2) -> (-147.2484, -128.9)
  line L9 (-147.2484, -128.9) -> (-17.2484, -128.9)
  line L10 (-17.2484, -128.9) -> (-17.2484, -129)
  line L11 (-17.2484, -129) -> (-70.0364, -129)
  line L12 (-70.0364, -129) -> (-70.0364, -130.5)
  line L13 (-70.0364, -130.5) -> (-70.0364, -132)
  line L14 (-70.0364, -132) -> (41.2244, -132)
  line L15 (41.2244, -132) -> (41.2244, -30)
  line L16 (41.2244, -30) -> (30.8999, -30)
  line L17 (30.8999, -30) -> (30.8999, -110)
  line L18 (30.8999, -110) -> (-61.0882, -110)
  line L19 (-61.0882, -110) -> (-61.0882, -30)
  line L20 (-61.0882, -30) -> (-70.2379, -30)
  line L21 (-70.2379, -30) -> (-70.0711, -104.5)
  line L22 (-70.0711, -104.5) -> (-70.0711, -113.1591)
  line L23 (-78, -139) -> (-84, -139)
  line L24 (-84, -139) -> (-84, -104)
  line L25 (-84, -104) -> (-78, -104)
  line L26 (-78, -104) -> (-78, -139)
  constraint horizontal L23
  constraint vertical L24
  constraint horizontal L25
  constraint vertical L26
extrude "Extrusion52" cut sketch "Skizze37" against normal blind 18 contours L7 L9 L24 L26 | L7 L24 L25 L26 | L9 L23 L24 L26 bodies 1 makes body 3 at (6.5654, 99.9556, 137.5)
extrude "Extrusion53" cut 1 faces at (78, 118.4333, 146.1) along direction (-1, 0, 0) blind 60.7 on bodies 3 bodies 3
sketch "Skizze38" plane through (0, 0, 147.5) normal (0, 0, 1) x (-1, 0, 0)
  line L0 (-84, -128.9) -> (-84, -113.2)
  line L1 (-84, -113.2) -> (-147.2484, -113.2)
  line L2 (-147.2484, -113.2) -> (-147.2484, -128.9)
  line L3 (-147.2484, -128.9) -> (-84, -128.9)
  line L4 (-147.2484, -114.8616) -> (-94.1484, -114.8616)
  line L5 (-94.1484, -107.782) -> (-83, -107.782)
  line L6 (-83, -107.782) -> (-83, -134)
  line L7 (-83, -134) -> (-94.1484, -134)
  line L8 (-94.1484, -134) -> (-94.1484, -107.782)
  dimension "d160" = 53.1
  constraint coincident L2 L4.start
  constraint perpendicular L2 L4
  constraint horizontal L5
  constraint vertical L6
  constraint horizontal L7
  constraint vertical L8
  measures "d160" distance of L4.start L4.end
extrude "Extrusion54" cut sketch "Skizze38" against normal blind 40 contours L0 L1 L3 L8 | L0 L1 L3 L5 L6 L7 L8 bodies 1
sketch "Skizze39" plane through (0, 0, 147.5) normal (0, 0, 1) x (-1, 0, 0)
  line L0 (-94.1484, -128.9) -> (-94.1484, -113.2)
  line L1 (-94.1484, -113.2) -> (-147.2484, -113.2)
  line L2 (-147.2484, -113.2) -> (-147.2484, -128.9)
  line L3 (-147.2484, -128.9) -> (-94.1484, -128.9)
  line L4 (-145, -116) -> (-144, -116)
  line L5 (-144, -116) -> (-144, -126)
  line L6 (-144, -126) -> (-145, -126)
  line L7 (-145, -126) -> (-145, -116)
  line L8 (-143, -117) -> (-142, -117)
  line L9 (-142, -117) -> (-142, -125)
  line L10 (-142, -125) -> (-143, -125)
  line L11 (-143, -125) -> (-143, -117)
  line L12 (-141, -118) -> (-140, -118)
  line L13 (-140, -118) -> (-140, -124)
  line L14 (-140, -124) -> (-141, -124)
  line L15 (-141, -124) -> (-141, -118)
  constraint horizontal L4
  constraint vertical L5
  constraint horizontal L6
  constraint vertical L7
  constraint horizontal L8
  constraint vertical L9
  constraint horizontal L10
  constraint vertical L11
  constraint horizontal L12
  constraint vertical L13
  constraint horizontal L14
  constraint vertical L15
extrude "Extrusion55" cut sketch "Skizze39" against normal blind 0.5 contours L4 L5 L6 L7 | L8 L9 L10 L11 | L12 L13 L14 L15 bodies 1
fillet "Abrundung5" radius 0.05 12 edges at (144, 121, 147.5) (142, 121, 147.5) (140, 121, 147.5) (140.5, 118, 147.5) (142.5, 117, 147.5) (144.5, 116, 147.5) (144.5, 126, 147.5) (142.5, 125, 147.5) (140.5, 124, 147.5) (141, 121, 147.5) (143, 121, 147.5) (145, 121, 147.5) on bodies 1
sketch "Skizze40" plane through (0, 0, 147.5) normal (0, 0, 1) x (-1, 0, 0)
  line L0 (-17.3, -113.2) -> (-17.3, -128.9)
  line L1 (-17.3, -128.9) -> (-17.2484, -128.9)
  line L2 (-17.2484, -128.9) -> (-17.2484, -129)
  line L3 (-17.2484, -129) -> (-70.0364, -129)
  line L4 (-70.0364, -129) -> (-70.0364, -130.5)
  line L5 (-70.0364, -130.5) -> (-70.0364, -132)
  line L6 (-70.0364, -132) -> (41.2244, -132)
  line L7 (41.2244, -132) -> (41.2244, -30)
  line L8 (41.2244, -30) -> (30.8999, -30)
  line L9 (30.8999, -30) -> (30.8999, -110)
  line L10 (30.8999, -110) -> (-61.0882, -110)
  line L11 (-61.0882, -110) -> (-61.0882, -30)
  line L12 (-61.0882, -30) -> (-70.2379, -30)
  line L13 (-70.2379, -30) -> (-70.0711, -104.5)
  line L14 (-70.0711, -104.5) -> (-70.0711, -113.1591)
  line L15 (-70.0711, -113.1591) -> (-17.2484, -113.1591)
  line L16 (-17.2484, -113.1591) -> (-17.2484, -113.2)
  line L17 (-17.2484, -113.2) -> (-17.3, -113.2)
  line L18 (25.1939, -122.719) -> (24, -120)
  line L19 (24, -120) -> (35.3869, -115)
  line L20 (35.3869, -115) -> (38.5, -115)
  line L21 (38.5, -115) -> (30.5, -122.719)
  line L22 (30.5, -122.719) -> (25.1939, -122.719)
  line L23 (19, -113) -> (39, -113)
  line L24 (39, -113) -> (39, -126)
  line L25 (39, -126) -> (19, -126)
  line L26 (19, -126) -> (19, -113)
  constraint horizontal L23
  constraint vertical L24
  constraint horizontal L25
  constraint vertical L26
extrude "Extrusion56" add sketch "Skizze40" against normal blind 1 contours L18 L19 L20 L21 L22 | L23 L24 L25 L26 bodies 3
sketch "Skizze41" plane through (0, 0, 147.5) normal (0, 0, 1) x (-1, 0, 0)
  line L0 (-17.3, -113.2) -> (-17.3, -128.9)
  line L1 (-17.3, -128.9) -> (-17.2484, -128.9)
  line L2 (-17.2484, -128.9) -> (-17.2484, -129)
  line L3 (-17.2484, -129) -> (-70.0364, -129)
  line L4 (-70.0364, -129) -> (-70.0364, -130.5)
  line L5 (-70.0364, -130.5) -> (-70.0364, -132)
  line L6 (-70.0364, -132) -> (41.2244, -132)
  line L7 (41.2244, -132) -> (41.2244, -30)
  line L8 (41.2244, -30) -> (30.8999, -30)
  line L9 (30.8999, -30) -> (30.8999, -110)
  line L10 (30.8999, -110) -> (-61.0882, -110)
  line L11 (-61.0882, -110) -> (-61.0882, -30)
  line L12 (-61.0882, -30) -> (-70.2379, -30)
  line L13 (-70.2379, -30) -> (-70.0711, -104.5)
  line L14 (-70.0711, -104.5) -> (-70.0711, -113.1591)
  line L15 (-70.0711, -113.1591) -> (-17.2484, -113.1591)
  line L16 (-17.2484, -113.1591) -> (-17.2484, -113.2)
  line L17 (-17.2484, -113.2) -> (-17.3, -113.2)
  line L18 (33.3256, -85.6956) -> (38.3923, -85.6956)
  line L19 (38.3923, -85.6956) -> (38.3923, -79.4967)
  line L20 (38.3923, -79.4967) -> (33.3256, -79.4967)
  line L21 (33.3256, -79.4967) -> (33.3256, -85.6956)
  constraint horizontal L18
  constraint vertical L19
  constraint horizontal L20
  constraint vertical L21
extrude "Extrusion57" cut sketch "Skizze41" against normal blind 5.8 contours L18 L19 L20 L21 bodies 3
sketch "Skizze42" plane through (-33.3256, 0, 0) normal (-1, 0, 0) x (0, -1, 0)
  line L0 (-85.6956, 146.1688) -> (-79.4967, 146.1688)
  line L1 (-79.4967, 146.1688) -> (-79.4967, 147.5)
  line L2 (-79.4967, 147.5) -> (-85.6956, 147.5)
  line L3 (-85.6956, 147.5) -> (-85.6956, 146.1688)
extrude "Extrusion58" add sketch "Skizze42" along normal blind 6 bodies 3
sketch "Skizze43" plane through (-41.2244, 0, 0) normal (-1, 0, 0) x (0, -1, 0)
  line L0 (-30, 147.5) -> (-132, 147.5)
  line L1 (-132, 147.5) -> (-132, 137.5)
  line L2 (-132, 137.5) -> (-30, 137.5)
  line L3 (-30, 137.5) -> (-30, 147.5)
  circle A0 centre (-82.7183, 143.5) radius 1.75
  line L4 (-84.573, 145.3877) -> (-71.373, 145.3877)
  line L5 (-71.373, 145.3877) -> (-71.373, 139.7877)
  line L6 (-71.373, 139.7877) -> (-84.573, 139.7877)
  line L7 (-84.573, 139.7877) -> (-84.573, 145.3877)
  dimension "d175" = 13.2
  dimension "d176" = 5.6
  constraint horizontal L4
  constraint vertical L5
  constraint horizontal L6
  constraint vertical L7
  measures "d175" distance of L4.start L4.end
  measures "d176" distance of L4.start L6.end
extrude "Extrusion59" add sketch "Skizze43" along normal blind 10 contours L0 L1 L2 L3 | L4 L5 L6 L7 bodies 3
sketch "Skizze44" plane through (-51.2244, 0, 0) normal (-1, 0, 0) x (0, -1, 0)
  circle A0 centre (-82.7183, 143.5) radius 1.75
  line L0 (-30, 137.5) -> (-30, 147.5)
  line L1 (-30, 147.5) -> (-132, 147.5)
  line L2 (-132, 147.5) -> (-132, 137.5)
  line L3 (-132, 137.5) -> (-30, 137.5)
  line L4 (-89.2292, 146) -> (-75.9892, 146)
  line L5 (-75.9892, 146) -> (-75.9892, 140.4)
  line L6 (-75.9892, 140.4) -> (-89.2292, 140.4)
  line L7 (-89.2292, 140.4) -> (-89.2292, 146)
  line L8 (-132, 147.5) -> (-91.9905, 147.5)
  line L9 (-91.9905, 147.5) -> (-91.9905, 137.5)
  line L10 (-91.9905, 137.5) -> (-132, 137.5)
  line L11 (-132, 137.5) -> (-132, 147.5)
  line L12 (-73.4478, 147.5) -> (-30, 147.5)
  line L13 (-30, 147.5) -> (-30, 137.5)
  line L14 (-30, 137.5) -> (-73.4478, 137.5)
  line L15 (-73.4478, 137.5) -> (-73.4478, 147.5)
  dimension "d179" = 13.24
  dimension "d180" = 5.6
  constraint horizontal L4
  constraint vertical L5
  constraint horizontal L6
  constraint vertical L7
  constraint horizontal L8
  constraint vertical L9
  constraint horizontal L10
  constraint vertical L11
  constraint coincident L3 L9.end
  constraint coincident L1.end L2.start
  constraint horizontal L12
  constraint vertical L13
  constraint horizontal L14
  constraint vertical L15
  constraint coincident L0.start L3.end
  measures "d179" distance of L4.start L4.end
  measures "d180" distance of L4.start L6.end
extrude "Extrusion60" cut sketch "Skizze44" against normal blind 10 contours L0 L1 L3 L12 L13 L14 L15 | L1 L2 L3 L8 L9 L10 L11 | L4 L5 L6 L7 bodies 3
extrude "Extrusion61" cut 1 faces at (-41.2244, 77.6489, 143.3) along direction (1, 0, 0) blind 8 on bodies 3 bodies 3
fillet "Abrundung6" radius 0.6 1 edges at (-38.5975, 89.2292, 142.9576) on bodies 3
fillet "Abrundung7" radius 0.75 1 edges at (17.2484, 119.681, 144.0424) on bodies 3
move_body "Verschieben16" bodies 2 to x (1, 0, 0) y (0, 1, 0) z (0, 0, 1) at (0, 0, 150)
sketch "Skizze45" plane through (0, 0, 149) normal (0, 0, 1) x (-1, 0, 0)
  line L0 (-60.2189, 96) -> (-60.2189, 16)
  line L1 (-60.2189, 16) -> (29.9888, 16)
  line L2 (29.9888, 16) -> (29.9888, 96)
  line L3 (29.9888, 96) -> (-60.2189, 96)
sketch "Skizze46" plane through (0, 0, 147.5) normal (0, 0, 1) x (-1, 0, 0)
  line L0 (41.2244, -132) -> (41.2244, -91.9905)
  line L1 (41.2244, -91.9905) -> (51.2244, -91.9905)
  line L2 (51.2244, -91.9905) -> (51.2244, -73.4478)
  line L3 (51.2244, -73.4478) -> (41.2244, -73.4478)
  line L4 (41.2244, -73.4478) -> (41.2244, -30)
  line L5 (41.2244, -30) -> (30.8999, -30)
  line L6 (30.8999, -30) -> (30.8999, -110)
  line L7 (30.8999, -110) -> (-61.0882, -110)
  line L8 (-61.0882, -110) -> (-61.0882, -30)
  line L9 (-61.0882, -30) -> (-70.2379, -30)
  line L10 (-70.2379, -30) -> (-70.0711, -104.5)
  line L11 (-70.0711, -104.5) -> (-70.0711, -113.1591)
  line L12 (-70.0711, -113.1591) -> (-17.2484, -113.1591)
  line L13 (-17.2484, -113.1591) -> (-17.2484, -113.2)
  line L14 (-17.2484, -113.2) -> (-17.3, -113.2)
  line L15 (-17.3, -113.2) -> (-17.3, -128.9)
  line L16 (-17.3, -128.9) -> (-17.2484, -128.9)
  line L17 (-17.2484, -128.9) -> (-17.2484, -129)
  line L18 (-17.2484, -129) -> (-70.0364, -129)
  line L19 (-70.0364, -129) -> (-70.0364, -130.5)
  line L20 (-70.0364, -130.5) -> (-70.0364, -132)
  line L21 (-70.0364, -132) -> (41.2244, -132)
sketch "Skizze47" plane through (67.2484, 0, 0) normal (-1, 0, 0) x (0, -1, 0)
  line L0 (-130.5, 147) -> (-130.5795, 147)
  line L1 (-130.5795, 147) -> (-130.5795, 139.5)
  line L2 (-130.5795, 139.5) -> (-111.5795, 139.5)
  line L3 (-111.5795, 139.5) -> (-111.5795, 147)
  line L4 (-111.5795, 147) -> (-111.6509, 147)
  line L5 (-111.6509, 147) -> (-111.6509, 145.6301)
  line L6 (-111.6509, 145.6301) -> (-130.5, 145.6301)
  line L7 (-130.5, 145.6301) -> (-130.5, 147)
  circle A0 centre (-114.5795, 142.2021) radius 2
  dimension "d190" = 4
  measures "d190" diameter of A0
extrude "Extrusion62" cut sketch "Skizze47" against normal blind 11 contours A0 bodies 3
fillet "Abrundung8" radius 0.05 2 edges at (67.2484, 116.4441, 142.9253) (70.044, 116.5795, 142.2021) on bodies 3
sketch "Skizze48" plane through (0, 0, 142.5) normal (0, 0, 1) x (-1, 0, 0)
  line L0 (-60.114, -110) -> (30.0937, -110)
  line L1 (30.0937, -110) -> (30.0937, -30)
  line L2 (30.0937, -30) -> (-60.114, -30)
  line L3 (-60.114, -30) -> (-60.114, -110)
  circle A0 centre (-40, -45) radius 6.5
  circle A1 centre (10, -45) radius 6.5
sketch "Skizze49" plane through (-51.2244, 0, 0) normal (-1, 0, 0) x (0, -1, 0)
  line L0 (-91.9905, 147.5) -> (-91.9905, 137.5)
  line L1 (-91.9905, 137.5) -> (-73.4478, 137.5)
  line L2 (-73.4478, 137.5) -> (-73.4478, 147.5)
  line L3 (-73.4478, 147.5) -> (-91.9905, 147.5)
  line L4 (-75.9892, 146) -> (-75.9892, 140.4)
  line L5 (-75.9892, 140.4) -> (-89.2292, 140.4)
  line L6 (-89.2292, 140.4) -> (-89.2292, 146)
  line L7 (-89.2292, 146) -> (-75.9892, 146)
  line L8 (-91.9905, 139.5193) -> (-73.1394, 139.5193)
  line L9 (-73.1394, 139.5193) -> (-73.1394, 138.1193)
  line L10 (-73.1394, 138.1193) -> (-91.9905, 138.1193)
  line L11 (-91.9905, 138.1193) -> (-91.9905, 139.5193)
  dimension "d195" = 1.4
  constraint horizontal L8
  constraint vertical L9
  constraint horizontal L10
  constraint vertical L11
  constraint coincident L0 L8.start
  measures "d195" distance of L8.start L10.end
extrude "Extrusion63" cut sketch "Skizze49" against normal blind 8 contours L0 L2 L8 L10 L11 | L2 L8 L9 L10 bodies 3
sketch "Skizze50" plane through (0, 91.9905, 0) normal (0, 1, 0) x (-1, 0, 0)
  line L0 (43.2244, 139.5193) -> (51.2244, 139.5193)
  line L1 (51.2244, 139.5193) -> (51.2244, 147.5)
  line L2 (51.2244, 147.5) -> (41.2244, 147.5)
  line L3 (41.2244, 147.5) -> (41.2244, 137.5)
  line L4 (41.2244, 137.5) -> (51.2244, 137.5)
  line L5 (51.2244, 137.5) -> (51.2244, 138.1193)
  line L6 (51.2244, 138.1193) -> (43.2244, 138.1193)
  line L7 (43.2244, 138.1193) -> (43.2244, 139.5193)
  line L8 (48.2244, 140) -> (51.2244, 140)
  line L9 (51.2244, 140) -> (51.2244, 137.5)
  line L10 (51.2244, 137.5) -> (48.2244, 137.5)
  line L11 (48.2244, 137.5) -> (48.2244, 140)
  constraint horizontal L8
  constraint vertical L9
  constraint horizontal L10
  constraint vertical L11
  constraint coincident L4.end L5.start
extrude "Extrusion64" add sketch "Skizze50" against normal blind 18.55 contours L0 L1 L8 L9 L11 | L0 L6 L9 L11 | L4 L5 L6 L9 L10 L11 bodies 3
sketch "Skizze51" plane through (0, 73.4405, 0) normal (0, -1, 0) x (1, 0, 0)
  line L0 (-51.2244, 137.5) -> (-48.2244, 137.5)
  line L1 (-48.2244, 137.5) -> (-48.2244, 140)
  line L2 (-48.2244, 140) -> (-51.2244, 140)
  line L3 (-51.2244, 140) -> (-51.2244, 137.5)
  line L4 (-51.2, 141.3) -> (-48.2244, 141.3)
  line L5 (-48.2244, 141.3) -> (-48.2244, 137.5)
  line L6 (-48.2244, 137.5) -> (-51.2, 137.5)
  line L7 (-51.2, 137.5) -> (-51.2, 141.3)
  constraint horizontal L4
  constraint vertical L5
  constraint horizontal L6
  constraint vertical L7
  constraint coincident L0.end L1.start
extrude "Extrusion65" add sketch "Skizze51" against normal blind 0.7 contours L0 L1 L2 L5 L6 L7 | L2 L4 L5 L7 bodies 3
extrude "Extrusion66" cut 1 faces at (-43.2244, 85.8096, 138.586) along direction (1, 0, 0) blind 1.6 on bodies 3 bodies 3
extrude "Extrusion67" add 1 faces at (-48.2244, 85.8096, 138.586) along direction (1, 0, 0) blind 1 on bodies 3 bodies 3
move_body "Verschieben17" bodies 1 to x (1, 0, 0) y (0, 1, 0) z (0, 0, 1) at (-77, 0, 0)
move_body "Verschieben18" bodies 1 to x (1, 0, 0) y (0, 1, 0) z (0, 0, 1) at (85, 0, 0)
sketch "Skizze52" plane through (0, 0, 147.5) normal (0, 0, 1) x (-1, 0, 0)
  line L0 (3.6661, -111.8642) -> (38.6661, -111.8642)
  line L1 (38.6661, -111.8642) -> (38.6661, -129.3642)
  line L2 (38.6661, -129.3642) -> (3.6661, -129.3642)
  line L3 (3.6661, -129.3642) -> (3.6661, -111.8642)
  dimension "d207" = 35
  dimension "d208" = 17.5
  constraint horizontal L0
  constraint vertical L1
  constraint horizontal L2
  constraint vertical L3
  measures "d207" distance of L0.start L0.end
  measures "d208" distance of L0.start L2.end
extrude "Extrusion68" cut sketch "Skizze52" against normal blind 8.5 bodies 3
move_body "Verschieben19" bodies 3 to x (1, 0, 0) y (0, 1, 0) z (0, 0, 1) at (0, 0, 45)
sketch "Skizze53" plane through (-3.6661, 0, 0) normal (-1, 0, 0) x (0, -1, 0)
  circle A0 centre (-121.0795, 188.5) radius 1.5
  line L0 (-111.8642, 192.5) -> (-129.3642, 192.5)
  line L1 (-129.3642, 192.5) -> (-129.3642, 184)
  line L2 (-129.3642, 184) -> (-111.8642, 184)
  line L3 (-111.8642, 184) -> (-111.8642, 192.5)
  line L4 (-129, 190) -> (-113, 190)
  line L5 (-113, 190) -> (-113, 187)
  line L6 (-113, 187) -> (-129, 187)
  line L7 (-129, 187) -> (-129, 190)
  constraint horizontal L4
  constraint vertical L5
  constraint horizontal L6
  constraint vertical L7
extrude "Extrusion69" cut sketch "Skizze53" against normal blind 22 contours A0 L4 L5 L6 | A0 L4 L6 L7 bodies 3
sketch "Skizze54" plane through (0, 0, 187) normal (0, 0, 1) x (-1, 0, 0)
  line L0 (-17.2484, -122.7565) -> (-17.2484, -129)
  line L1 (-17.2484, -129) -> (3.6661, -129)
  line L2 (3.6661, -129) -> (3.6661, -113)
  line L3 (3.6661, -113) -> (-17.2484, -113)
  line L4 (-17.2484, -113) -> (-17.2484, -119.4024)
  spline S0 degree 3 poles (-16.4984, -121.0795) (-16.5117, -121.0606) (-16.525, -121.0417) (-16.7821, -120.678) (-16.9909, -120.3646) (-17.1853, -119.8615) (-17.2311, -119.6857) (-17.247, -119.4721) (-17.2484, -119.4372) (-17.2484, -119.4024) knots -0.239149 -0.239149 -0.239149 -0.239149 -0.233316 -0.233316 -0.126855 -0.126855 -0.073449 -0.073449 -0.063061 -0.063061 -0.063061 -0.063061
  spline S1 degree 3 poles (-17.2484, -122.7565) (-17.2484, -122.7218) (-17.247, -122.687) (-17.2311, -122.4735) (-17.1854, -122.2977) (-16.9911, -121.7946) (-16.7822, -121.4811) (-16.5253, -121.1177) (-16.5122, -121.0991) (-16.4991, -121.0806) knots -0.202547 -0.202547 -0.202547 -0.202547 -0.190208 -0.190208 -0.126696 -0.126696 0 0 0.006807 0.006807 0.006807 0.006807
  line L5 (3.6661, -122.5799) -> (1.5, -122.5799)
  line L6 (1.5, -122.5799) -> (1.5, -120)
  line L7 (1.5, -120) -> (3.6661, -120)
  line L8 (3.6661, -120) -> (3.6661, -122.5799)
  constraint horizontal L5
  constraint vertical L6
  constraint horizontal L7
  constraint vertical L8
  constraint coincident L2 L5.start
extrude "Extrusion70" add sketch "Skizze54" along normal blind 3 contours L2 L5 L6 L7 L8 bodies 3
extrude "Extrusion71" add 1 faces at (-1.5, 121.7199, 188) along direction (1, 0, 0) blind 19 on bodies 3 bodies 3
sketch "Skizze55" plane through (17.2484, 0, 0) normal (1, 0, 0) x (0, 1, 0)
  line L0 (122.7565, 190) -> (129, 190)
  line L1 (129, 190) -> (129, 187)
  line L2 (129, 187) -> (122.7565, 187)
  arc A0 (119.4024, 187) -> (122.7565, 187) centre (121.0795, 188.5) ccw
  line L3 (119.4024, 187) -> (113, 187)
  line L4 (113, 187) -> (113, 190)
  line L5 (113, 190) -> (119.4024, 190)
  arc A1 (120.6078, 190.7) -> (119.4024, 190) centre (121.0795, 188.5) ccw
  line L6 (120.6078, 190.7) -> (111.7, 190.7)
  line L7 (111.7, 190.7) -> (111.7, 191.9)
  line L8 (111.7, 191.9) -> (113.2, 191.9)
  line L9 (113.2, 191.9) -> (113.2, 192.5)
  line L10 (113.2, 192.5) -> (113.1591, 192.5)
  line L11 (113.1591, 192.5) -> (113.1591, 192)
  line L12 (113.1591, 192) -> (111.5795, 192)
  line L13 (111.5795, 192) -> (111.5795, 184.5)
  line L14 (111.5795, 184.5) -> (130.5795, 184.5)
  line L15 (130.5795, 184.5) -> (130.5795, 192)
  line L16 (130.5795, 192) -> (129, 192)
  line L17 (129, 192) -> (129, 192.5)
  line L18 (129, 192.5) -> (128.9, 192.5)
  line L19 (128.9, 192.5) -> (128.9, 191.9)
  line L20 (128.9, 191.9) -> (130.4, 191.9)
  line L21 (130.4, 191.9) -> (130.4, 190.7)
  line L22 (130.4, 190.7) -> (121.5512, 190.7)
  arc A2 (122.7565, 190) -> (121.5512, 190.7) centre (121.0795, 188.5) ccw
  line L23 (129.5, 184.5) -> (111.5795, 184.5)
  line L24 (111.5795, 184.5) -> (111.5795, 190.7)
  line L25 (111.5795, 190.7) -> (129.5, 190.7)
  line L26 (129.5, 190.7) -> (129.5, 184.5)
  constraint horizontal L23
  constraint vertical L24
  constraint horizontal L25
  constraint vertical L26
  constraint coincident L13 L24.end
  constraint coincident L14 L23.start
extrude "Extrusion73" cut 1 faces at (17.5, 121.7199, 188) along direction (-1, 0, 0) blind 0.5 on bodies 3 bodies 3